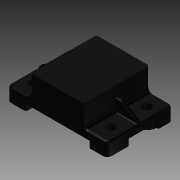
# Autodesk Inventor part: BUSS-BASE
Saved by Autodesk Inventor 2014 SP1 (Build 180222100, 222)
## iProperties
Shininess: 64.0
Length Units: 11272
Angle Units: 11279
Time Units: 11290
Mass Units: 11286
Length Display Precision: 3
Angle Display Precision: 2
Compacted: True
Part Number: BUSS-BASE
Document SubType Name: Modeling
Created: 2003-01-10
Designer: geyerm
Density: 1 g/cm^3
Material: Generic
Mass: 50.4204 g
Surface Area: 132.632 cm^2
Volume: 50.4204 cm^3
Appearance: Glossy - Black
Density: 0.0
Volumn: 0.0
Area: 0.0
PropertySet Name: Model Information
Control State: 0
Master: False
Checked Out: False
Author: Autodesk
Autodesk Inventor part; units mm, degrees
ref_plane "YZ Plane" through (0, 0, 0) normal (1, 0, 0) x (0, 1, 0)
ref_plane "XZ Plane" through (0, 0, 0) normal (0, 1, 0) x (-1, 0, 0)
ref_plane "XY Plane" through (0, 0, 0) normal (0, 0, 1) x (1, 0, 0)
sketch "Sketch1" plane through (0, 0, 0) normal (0, 0, 1) x (1, 0, 0)
  line L0 (-36.83, 0) -> (36.83, 0)
  line L1 (36.83, 0) -> (36.83, 5.08)
  line L2 (36.83, 5.08) -> (-36.83, 5.08)
  line L3 (-36.83, 5.08) -> (-36.83, 0)
  line L4 (-19.431, 5.08) -> (19.431, 5.08)
  line L5 (19.431, 5.08) -> (19.431, 21.336)
  line L6 (19.431, 21.336) -> (-19.431, 21.336)
  line L7 (-19.431, 21.336) -> (-19.431, 5.08)
  line L8 (0, 0) -> (0, 46.386) construction
  dimension "d1" = 21.336
  dimension "d2" = 5.08
  dimension "d3" = 73.66
  dimension "d4" = 38.862
  constraints: 18 end point, 5 parallel, 2 horizontal, 2 perpendicular, 1 midpoint, 1 point on line, 1 vertical, 3 other
  measures "d1" distance between parallel lines of L6 L0
  measures "d2" distance of L2.end L0.start
  measures "d3" distance of L0.start L0.end
  measures "d4" distance of L5.end L6.end
extrude "Extrusion1" add sketch "Sketch1" along normal mid plane 48.26
fillet "Fillet19" radius 3.048 2 edges at (19.431, 5.08, 0) (-19.431, 5.08, 0)
ref_plane "Work Plane6" through (0, 0, 0) normal (0, 0, 1) x (1, 0, 0)
ref_plane "Work Plane7" through (0, 0, 24.13) normal (1, 0, 0) x (0, 0, -1)
sketch "Sketch5" plane through (36.83, 5.08, 24.13) normal (0, 1, 0) x (1, 0, 0)
  circle A0 centre (-8.509, 37.465) radius 3.302
  line L0 (15.3553, 24.13) -> (-89.0153, 24.13) projected
  line L1 (-36.83, 57.912) -> (-36.83, -9.652) projected
  dimension "d43" = 6.604
  dimension "d127" = 13.335
  dimension "d128" = 28.321
  constraints: 1 centre point
  measures "d43" diameter of A0
  measures "d127" distance from line of A0.centre L0
  measures "d128" distance from line of A0.centre L1
extrude "Extrusion4" cut sketch "Sketch5" against normal through all
fillet "Fillet20" radius 3.048 4 edges at (-36.83, 2.54, 24.13) (36.83, 2.54, 24.13) (36.83, 2.54, -24.13) (-36.83, 2.54, -24.13)
sketch "Sketch14" plane through (-33.782, 0, 24.13) normal (0, -1, 0) x (1, 0, 0)
  line L0 (70.612, -45.212) -> (70.612, -3.048) projected
  line L1 (67.564, 0) -> (0, 0) projected
  line L2 (0, -48.26) -> (67.564, -48.26) projected
  line L3 (56.9825, -2.4842) -> (67.9045, -15.9462)
  line L4 (70.612, -14.986) -> (70.612, -3.048)
  line L5 (67.564, 0) -> (58.166, 0)
  arc A0 (70.612, -3.048) -> (67.564, 0) centre (67.564, -3.048) ccw
  arc A1 (58.166, 0) -> (56.9825, -2.4842) centre (58.166, -1.524) ccw
  arc A2 (67.9045, -15.9462) -> (70.612, -14.986) centre (69.088, -14.986) ccw
  dimension "d83" = 3.048
  dimension "d84" = 1.524
  dimension "d85" = 13.97
  dimension "d86" = 16.51
  constraints: 6 end point, 6 point on circle, 6 tangent, 3 centre point, 2 collinear, 1 equal radius, 1 parallel
  measures "d83" radius of A0
  measures "d84" radius of A1
extrude "Extrusion10" add sketch "Sketch14" along normal blind 4.826
sketch "Sketch16" plane through (-33.782, 0, -24.13) normal (0, -1, 0) x (1, 0, 0)
  line L0 (-3.048, 45.212) -> (-3.048, 3.048) projected
  line L1 (0, 0) -> (67.564, 0) projected
  line L2 (70.612, 3.048) -> (70.612, 33.274) projected
  line L3 (-0.3405, 15.9462) -> (10.5815, 2.4842)
  line L4 (9.398, 0) -> (0, 0)
  line L5 (-3.048, 3.048) -> (-3.048, 14.986)
  arc A0 (-3.048, 3.048) -> (0, 0) centre (0, 3.048) ccw
  arc A1 (-0.3405, 15.9462) -> (-3.048, 14.986) centre (-1.524, 14.986) ccw
  arc A2 (9.398, 0) -> (10.5815, 2.4842) centre (9.398, 1.524) ccw
  dimension "d92" = 3.048
  dimension "d93" = 1.524
  dimension "d94" = 16.51
  dimension "d95" = 13.97
  constraints: 6 end point, 6 point on circle, 6 tangent, 3 centre point, 2 collinear, 2 perpendicular, 1 equal radius
  measures "d92" radius of A0
  measures "d93" radius of A1
extrude "Extrusion12" add sketch "Sketch16" along normal blind 4.826
fillet "Fillet21" radius 1.524 18 edges at (-19.431, 14.732, 24.13) (-20.3237, 5.9727, 24.13) (-28.1305, 5.08, 24.13) (-35.9373, 5.08, 23.2373) (-36.83, 5.08, 0) (-35.9373, 5.08, -23.2373) (-28.1305, 5.08, -24.13) (-20.3237, 5.9727, -24.13) (-19.431, 14.732, -24.13) (19.431, 14.732, 24.13) (20.3237, 5.9727, 24.13) (28.1305, 5.08, 24.13) (35.9373, 5.08, 23.2373) (36.83, 5.08, 0) (35.9373, 5.08, -23.2373) (28.1305, 5.08, -24.13) (20.3237, 5.9727, -24.13) (19.431, 14.732, -24.13)
ref_plane "Work Plane3" through (36.83, 0, 0) normal (0, 0, 1) x (1, 0, 0)
ref_plane "Work Plane4" through (0, 0, 24.13) normal (-1, 0, 0) x (0, -1, 0)
mirror "Mirror4" about plane through (36.83, 0, 0) normal (0, 0, 1) of "Extrusion4"
mirror "Mirror5" about plane through (0, 0, 24.13) normal (-1, 0, 0) of "Extrusion4", "Mirror4"
sketch "Sketch15" plane through (-33.782, -4.826, 24.13) normal (0, -1, 0) x (1, 0, 0)
  arc A0 (65.0043, -12.3715) -> (61.1583, -7.631) centre (62.103, -10.795) ccw projected
  arc A1 (67.9045, -15.9462) -> (70.612, -14.986) centre (69.088, -14.986) ccw projected
  line L0 (70.612, -3.048) -> (70.612, -14.986) projected
  arc A2 (70.612, -3.048) -> (67.564, 0) centre (67.564, -3.048) ccw projected
  line L1 (58.166, 0) -> (67.564, 0) projected
  arc A3 (58.166, 0) -> (56.9825, -2.4842) centre (58.166, -1.524) ccw projected
  line L2 (61.1583, -7.631) -> (56.9825, -2.4842) projected
  arc A4 (58.166, -1.27) -> (57.9688, -1.684) centre (58.166, -1.524) ccw
  line L3 (58.166, -1.27) -> (67.564, -1.27)
  arc A5 (69.342, -3.048) -> (67.564, -1.27) centre (67.564, -3.048) ccw
  line L4 (69.342, -3.048) -> (69.342, -14.986)
  arc A6 (68.8908, -15.146) -> (69.342, -14.986) centre (69.088, -14.986) ccw
  line L5 (68.8908, -15.146) -> (65.2252, -11.8699)
  line L6 (61.6947, -7.5183) -> (57.9688, -1.684)
  arc A7 (61.6947, -7.5183) -> (61.1583, -7.631) centre (62.103, -10.795) ccw
  arc A8 (65.0043, -12.3715) -> (65.2252, -11.8699) centre (62.103, -10.795) ccw
  dimension "d89" = 1.27
  constraints: 13 point on circle, 9 end point, 5 centre point, 1 coincident, 4 other
  measures "d89" distance between parallel lines of L1 L3
extrude "Extrusion11" cut sketch "Sketch15" against normal up to surface (4.826 mm away)
sketch "Sketch17" plane through (-33.782, -4.826, -24.13) normal (0, -1, 0) x (1, 0, 0)
  arc A0 (2.5597, 12.3715) -> (6.4057, 7.631) centre (5.461, 10.795) ccw projected
  line L0 (-0.3405, 15.9462) -> (2.5597, 12.3715) projected
  arc A1 (-0.3405, 15.9462) -> (-3.048, 14.986) centre (-1.524, 14.986) ccw projected
  line L1 (-3.048, 3.048) -> (-3.048, 14.986) projected
  arc A2 (-3.048, 3.048) -> (0, 0) centre (0, 3.048) ccw projected
  line L2 (9.398, 0) -> (0, 0) projected
  arc A3 (9.398, 0) -> (10.5815, 2.4842) centre (9.398, 1.524) ccw projected
  line L3 (6.4057, 7.631) -> (10.5815, 2.4842) projected
  arc A4 (-1.3268, 15.146) -> (-1.778, 14.986) centre (-1.524, 14.986) ccw
  line L4 (-1.3268, 15.146) -> (2.2973, 11.7408)
  line L5 (5.7345, 7.5043) -> (9.5952, 1.684)
  arc A5 (9.398, 1.27) -> (9.5952, 1.684) centre (9.398, 1.524) ccw
  line L6 (9.398, 1.27) -> (0, 1.27)
  arc A6 (-1.778, 3.048) -> (0, 1.27) centre (0, 3.048) ccw
  line L7 (-1.778, 3.048) -> (-1.778, 14.986)
  arc A7 (2.5597, 12.3715) -> (2.2973, 11.7408) centre (5.461, 10.795) ccw
  arc A8 (5.7345, 7.5043) -> (6.4057, 7.631) centre (5.461, 10.795) ccw
  dimension "d98" = 1.27
  constraints: 10 end point, 10 point on circle, 5 centre point, 1 coincident, 3 other
  measures "d98" distance between parallel lines of L1 L7
extrude "Extrusion13" cut sketch "Sketch17" against normal up to surface (4.826 mm away) contours A0 L5 A5 L6 A6 L7 A4 L4
sketch "Sketch18" plane through (-33.782, 0, 24.13) normal (0, -1, 0) x (1, 0, 0)
  circle A0 centre (5.461, -10.795) radius 3.302 projected
  line L0 (9.398, -48.26) -> (67.564, -48.26) projected
  line L1 (70.612, -45.212) -> (70.612, -14.986) projected
  line L2 (58.166, 0) -> (0, 0) projected
  line L3 (-3.048, -3.048) -> (-3.048, -33.274) projected
  circle A1 centre (62.103, -37.465) radius 3.302 projected
  circle A2 centre (5.461, -10.795) radius 6.985
  circle A3 centre (62.103, -37.465) radius 6.985
  line L4 (-1.524, -10.795) -> (-2.032, -10.795)
  line L5 (-3.048, -9.779) -> (-3.048, -3.048)
  line L6 (0, 0) -> (9.398, 0)
  line L7 (10.922, -1.524) -> (10.922, -6.4398)
  arc A4 (0, 0) -> (-3.048, -3.048) centre (0, -3.048) ccw
  arc A5 (10.922, -1.524) -> (9.398, 0) centre (9.398, -1.524) ccw
  arc A6 (-3.048, -9.779) -> (-2.032, -10.795) centre (-2.032, -9.779) ccw
  line L8 (69.088, -37.465) -> (69.596, -37.465)
  line L9 (70.612, -38.481) -> (70.612, -45.212)
  line L10 (67.564, -48.26) -> (58.166, -48.26)
  line L11 (56.642, -46.736) -> (56.642, -41.8202)
  arc A7 (67.564, -48.26) -> (70.612, -45.212) centre (67.564, -45.212) ccw
  arc A8 (56.642, -46.736) -> (58.166, -48.26) centre (58.166, -46.736) ccw
  arc A9 (70.612, -38.481) -> (69.596, -37.465) centre (69.596, -38.481) ccw
  dimension "d101" = 13.97
  dimension "d102" = 13.97
  dimension "d103" = 3.048
  dimension "d104" = 1.524
  dimension "d105" = 1.016
  dimension "d106" = 3.048
  dimension "d107" = 1.524
  dimension "d108" = 1.016
  dimension "d109" = 13.97
  constraints: 16 end point, 16 point on circle, 12 tangent, 8 centre point, 4 collinear, 4 parallel, 4 perpendicular, 2 coincident, 2 concentric, 2 point on line, 1 equal radius
  measures "d101" diameter of A2
  measures "d102" distance between parallel lines of L7 L5
  measures "d103" radius of A4
  measures "d104" radius of A5
  measures "d105" radius of A6
  measures "d106" radius of A7
  measures "d107" radius of A8
  measures "d108" radius of A9
  measures "d109" distance between parallel lines of L9 L11
extrude "Extrusion14" add sketch "Sketch18" along normal blind 4.826
sketch "Sketch19" plane through (-33.782, -4.826, 24.13) normal (0, -1, 0) x (1, 0, 0)
  circle A0 centre (5.461, -10.795) radius 3.302 projected
  arc A1 (-1.524, -10.795) -> (10.922, -6.4398) centre (5.461, -10.795) ccw projected
  arc A2 (10.922, -1.524) -> (9.398, 0) centre (9.398, -1.524) ccw projected
  line L0 (0, 0) -> (9.398, 0) projected
  arc A3 (0, 0) -> (-3.048, -3.048) centre (0, -3.048) ccw projected
  line L1 (-3.048, -9.779) -> (-3.048, -3.048) projected
  arc A4 (9.0739, -4.817) -> (-1.0423, -8.246) centre (5.461, -10.795) ccw
  line L2 (9.652, -4.4909) -> (9.652, -1.524)
  line L3 (9.398, -1.27) -> (0, -1.27)
  line L4 (-1.778, -3.048) -> (-1.778, -8.1069)
  arc A5 (0, -1.27) -> (-1.778, -3.048) centre (0, -3.048) ccw
  arc A6 (1.1694, -5.2839) -> (1.7128, -4.9008) centre (0, -3.048) ccw
  arc A7 (9.652, -1.524) -> (9.398, -1.27) centre (9.398, -1.524) ccw
  arc A8 (-1.778, -8.1069) -> (-1.0423, -8.246) centre (-1.397, -8.1069) ccw
  arc A9 (9.0739, -4.817) -> (9.652, -4.4909) centre (9.271, -4.4909) ccw
  dimension "d112" = 1.27
  dimension "d113" = 1.27
  dimension "d114" = 0.381
  dimension "d116" = 0.381
  dimension "d117" = 13.97
  constraints: 15 point on circle, 8 tangent, 6 centre point, 6 end point, 3 coincident, 2 concentric, 2 parallel, 1 perpendicular
  measures "d112" distance between parallel lines of L0 L3
  measures "d113" distance between parallel lines of L1 L4
  measures "d114" radius of A8
  measures "d116" radius of A9
  measures "d117" diameter of A4
extrude "Extrusion15" cut sketch "Sketch19" against normal up to surface (4.826 mm away) contours A4 A8 L4 A5 L3 A7 L2 A9
sketch "Sketch20" plane through (-33.782, -4.826, 24.13) normal (0, -1, 0) x (1, 0, 0)
  circle A0 centre (62.103, -37.465) radius 3.302 projected
  arc A1 (69.088, -37.465) -> (56.642, -41.8202) centre (62.103, -37.465) ccw projected
  line L0 (56.642, -46.736) -> (56.642, -41.8202) projected
  arc A2 (56.642, -46.736) -> (58.166, -48.26) centre (58.166, -46.736) ccw projected
  arc A3 (67.564, -48.26) -> (70.612, -45.212) centre (67.564, -45.212) ccw projected
  line L1 (70.612, -38.481) -> (70.612, -45.212) projected
  arc A4 (58.4901, -43.443) -> (68.6063, -40.014) centre (62.103, -37.465) ccw
  line L2 (57.912, -43.7691) -> (57.912, -46.736)
  line L3 (58.166, -46.99) -> (67.564, -46.99)
  line L4 (69.342, -45.212) -> (69.342, -40.1531)
  arc A5 (67.564, -46.99) -> (69.342, -45.212) centre (67.564, -45.212) ccw
  arc A6 (57.912, -46.736) -> (58.166, -46.99) centre (58.166, -46.736) ccw
  arc A7 (69.342, -40.1531) -> (68.6063, -40.014) centre (68.961, -40.1531) ccw
  arc A8 (58.4901, -43.443) -> (57.912, -43.7691) centre (58.293, -43.7691) ccw
  dimension "d120" = 1.27
  dimension "d121" = 0.381
  dimension "d122" = 0.381
  dimension "d124" = 13.97
  constraints: 11 point on circle, 8 end point, 8 tangent, 5 centre point, 3 coincident, 2 concentric, 2 parallel, 1 perpendicular
  measures "d120" distance between parallel lines of L1 L4
  measures "d121" radius of A7
  measures "d122" radius of A8
  measures "d124" diameter of A4
extrude "Extrusion16" cut sketch "Sketch20" against normal up to surface (4.826 mm away) contours A4 A7 L4 A5 L3 A6 L2 A8
sketch "Sketch6" plane through (22.479, 5.08, -22.606) normal (0, 1, 0) x (1, 0, 0)
  circle A0 centre (5.842, -35.941) radius 3.302 projected
  line L0 (0, -45.212) -> (0, 0) projected
  line L1 (12.827, -1.524) -> (12.827, -43.688) projected
  line L2 (0, -28.956) -> (5.842, -28.956)
  arc A1 (5.842, -42.926) -> (5.842, -28.956) centre (5.842, -35.941) ccw
  line L3 (5.842, -42.926) -> (0, -42.926)
  line L4 (0, -42.926) -> (0, -28.956)
  constraints: 6 end point, 3 tangent, 2 perpendicular, 2 point on circle, 1 centre point, 1 collinear, 1 concentric, 1 parallel
extrude "Extrusion5" add sketch "Sketch6" along normal blind 0.381
sketch "Sketch7" plane through (-33.782, 5.08, -22.606) normal (0, 1, 0) x (1, 0, 0)
  circle A0 centre (5.461, -9.271) radius 3.302 projected
  line L0 (-1.524, -43.688) -> (-1.524, -1.524) projected
  line L1 (11.303, 0) -> (11.303, -45.212) projected
  line L2 (11.303, -2.286) -> (5.461, -2.286)
  arc A1 (5.461, -2.286) -> (5.461, -16.256) centre (5.461, -9.271) ccw
  line L3 (5.461, -16.256) -> (11.303, -16.256)
  line L4 (11.303, -16.256) -> (11.303, -2.286)
  constraints: 6 end point, 3 tangent, 2 perpendicular, 2 point on circle, 1 centre point, 1 collinear, 1 concentric, 1 parallel
extrude "Extrusion6" add sketch "Sketch7" along normal blind 0.381
sketch "Sketch8" plane through (36.83, 0, 0) normal (0, 0, 1) x (1, 0, 0)
  line L0 (-56.261, 23.099) -> (-17.399, 23.099) projected
  line L1 (-17.399, 23.099) -> (-17.399, 8.128) projected
  arc A0 (-17.399, 8.128) -> (-14.351, 5.08) centre (-14.351, 8.128) ccw projected
  line L2 (-14.351, 5.08) -> (-1.524, 5.08) projected
  arc A1 (0, 3.556) -> (-1.524, 5.08) centre (-1.524, 3.556) ccw projected
  line L3 (0, 3.556) -> (0, 0) projected
  line L4 (0, 0) -> (-73.66, 0) projected
  line L5 (-73.66, 0) -> (-73.66, 3.556) projected
  arc A2 (-72.136, 5.08) -> (-73.66, 3.556) centre (-72.136, 3.556) ccw projected
  line L6 (-72.136, 5.08) -> (-59.309, 5.08) projected
  arc A3 (-59.309, 5.08) -> (-56.261, 8.128) centre (-59.309, 8.128) ccw projected
  line L7 (-56.261, 8.128) -> (-56.261, 23.099) projected
  line L8 (-16.1943, 13.716) -> (-14.097, 13.716)
  line L9 (-12.3995, 13.2463) -> (-1.5831, 6.7636)
  arc A4 (0, 3.556) -> (-1.5831, 6.7636) centre (-3.2806, 3.9314) ccw
  arc A5 (-12.3995, 13.2463) -> (-14.097, 13.716) centre (-14.097, 10.414) ccw
  dimension "d52" = 3.302
  dimension "d53" = 3.302
  dimension "d54" = 8.636
  dimension "d55" = 3.302
  constraints: 4 end point, 4 point on circle, 3 tangent, 2 centre point, 1 parallel, 1 perpendicular
  measures "d52" radius of A4
  measures "d53" radius of A5
  measures "d54" distance between parallel lines of L8 L2
  measures "d55" distance from line of A5.centre L1
extrude "Rib2" add sketch "Sketch8" along normal mid plane 2.54 rib yes fills toward (-15.1456, 13.666) open curves L8 A5 L9 A4
fillet "Fillet22" radius 0.762 8 edges at (29.8387, 10.005, 1.27) (36.5104, 5.3928, 1.27) (23.6136, 13.5964, 1.27) (21.082, 13.716, 1.27) (29.8387, 10.005, -1.27) (23.6136, 13.5964, -1.27) (21.082, 13.716, -1.27) (36.5104, 5.3928, -1.27)
fillet "Fillet23" radius 0.762 14 edges at (19.431, 10.541, 1.27) (19.431, 13.4928, 1.0468) (19.431, 13.716, 0) (19.431, 13.4928, -1.0468) (19.431, 10.541, -1.27) (20.3237, 5.9727, -1.27) (28.8925, 5.08, -1.27) (35.5909, 5.0531, -1.27) (36.6106, 4.3438, -1.0366) (36.83, 3.556, 0) (36.6105, 4.3439, 1.0366) (35.5909, 5.0531, 1.27) (28.8925, 5.08, 1.27) (20.3237, 5.9727, 1.27)
mirror "Mirror6" about plane through (0, 0, 24.13) normal (-1, 0, 0) of "Rib2", "Fillet22", "Fillet23"
equation "\"d92\" = d83"
equation "\"d94\" = d86"
equation "\"d95\" = d85"
equation "\"d96\" = d87"
equation "\"d98\" = d89"
equation "\"d99\" = d87"
equation "\"d103\" = d83"
equation "\"d106\" = d103"
equation "\"d109\" = d102"
equation "\"d110\" = d87"
equation "\"d116\" = d114"
equation "\"d118\" = d87"
equation "\"d120\" = d112"
equation "\"d121\" = d114"
equation "\"d122\" = d121"
equation "\"d125\" = d87"
equation "\"d87\" = 4.826"
body "Solid1"
